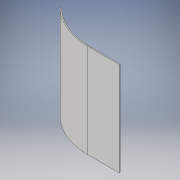
# Autodesk Inventor part: Hood.ver1-1111-2020
Saved by Autodesk Inventor 2018 (Build 220112000, 112)
## iProperties
Created: 2020-01-19
Part Number: Hood.ver1-1111-2020
Material: Generic
Document SubType Name: Modeling
Designer: JMHal
Density: 1 g/cm^3
Appearance: Default
Author: JMHal
Autodesk Inventor part; units mm, degrees
ref_plane "YZ Plane" through (0, 0, 0) normal (1, 0, 0) x (0, 1, 0)
ref_plane "XZ Plane" through (0, 0, 0) normal (0, 1, 0) x (-1, 0, 0)
ref_plane "XY Plane" through (0, 0, 0) normal (0, 0, 1) x (1, 0, 0)
sketch "Sketch1" plane through (0, 0, 0) normal (0, 1, 0) x (-1, 0, 0)
  circle A0 centre (0, 0) radius 215.9
  circle A1 centre (0, 0) radius 219.075
  line L0 (0, 219.075) -> (-101.6, 219.075)
  line L1 (-101.6, 219.075) -> (-101.6, 215.9)
  line L2 (-101.6, 215.9) -> (0, 215.9)
  line L3 (0, 0) -> (0, 219.075)
  line L4 (0, 0) -> (154.9094, 154.9094)
  line L5 (-101.6, 215.9) -> (0, 215.9)
  line L6 (0, 215.9) -> (0, 219.075)
  line L7 (0, 219.075) -> (-101.6, 219.075)
  line L8 (-101.6, 219.075) -> (-101.6, 215.9)
  arc A2 (152.6644, 152.6644) -> (0, 215.9) centre (0, 0) ccw
  arc A3 (154.9094, 154.9094) -> (0, 219.075) centre (0, 0) ccw
  dimension "d0" = 431.8
  dimension "d1" = 3.175
  dimension "d2" = 101.6
  dimension "d3" = 3.175
  dimension "d4" = 45
  constraints: 18 end point, 8 point on circle, 4 centre point, 3 perpendicular, 3 tangent, 2 horizontal, 2 parallel, 1 coincident, 1 point on line, 1 vertical
  measures "d0" diameter of A0
  measures "d1" radial gap between concentric circles of A0 A1
  measures "d2" distance of L0.start L0.end
  measures "d3" distance of L0.end L1.end
  measures "d4" angle of L3 L4
extrude "Extrusion1" add sketch "Sketch1" along normal blind 304.8 contours A0 L3 A1 L4 | L2 A1 L3 | L2 L1 L0 A1
body "Solid1"
